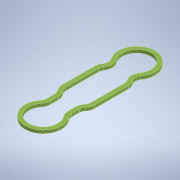
# Autodesk Inventor part: Base Seal
Saved by Autodesk Inventor 2021 (Build 250183000, 183)
## iProperties
Created: 2020-06-02
Part Number: Base Seal
Material: Generic
Document SubType Name: Modeling
Designer: jgray
Density: 1 g/cm^3
Appearance: Default
Author: jgray
Autodesk Inventor part; units mm, degrees
ref_plane "YZ Plane" through (0, 0, 0) normal (1, 0, 0) x (0, 1, 0)
ref_plane "XZ Plane" through (0, 0, 0) normal (0, 1, 0) x (-1, 0, 0)
ref_plane "XY Plane" through (0, 0, 0) normal (0, 0, 1) x (1, 0, 0)
sketch "Sketch1" plane through (0, 0, 0) normal (0, 1, 0) x (-1, 0, 0)
  line L0 (13.9, 33.875) -> (-13.9, 33.875)
  line L1 (-13.9, 33.875) -> (-13.9, -33.875)
  line L2 (-13.9, -33.875) -> (13.9, -33.875)
  line L3 (13.9, -33.875) -> (13.9, 33.875)
  circle A0 centre (9.4, 30.5) radius 1.7
  circle A1 centre (-9.4, 15) radius 1.7
  circle A2 centre (9.4, -15) radius 1.7
  circle A3 centre (-9.4, -15) radius 1.7
  circle A4 centre (-9.4, -30.5) radius 1.7
  circle A5 centre (9.4, -30.5) radius 1.7
  circle A6 centre (9.4, 15) radius 1.7
  circle A7 centre (-9.4, 30.5) radius 1.7
  arc A8 (-3.4662, -17.8593) -> (3.4662, -17.8593) centre (0, -22) ccw
  line L4 (4.7, 5.1) -> (4.7, -10.1)
  arc A9 (2.75, -12.0994) -> (4.7, -10.1) centre (2.7, -10.1) ccw
  arc A10 (-4.7, -10.1) -> (-2.75, -12.0994) centre (-2.7, -10.1) ccw
  line L5 (-4.7, -10.1) -> (-4.7, 5.1)
  line L6 (-2.75, 7.0994) -> (-2.75, 16.3257)
  arc A11 (3.4662, 17.8593) -> (-3.4662, 17.8593) centre (0, 22) ccw
  line L7 (2.75, -12.0994) -> (2.75, -16.3257)
  arc A12 (-5.2039, -18.2745) -> (5.2039, -18.2745) centre (0, -22) ccw
  line L8 (-3.75, 14.4782) -> (-3.75, 11.1034)
  arc A13 (-5.0936, 7.4643) -> (-5.7, 5.8219) centre (-3.1726, 5.8219) ccw
  arc A14 (-5.7, -10.1) -> (-5.1619, -11.8144) centre (-2.7, -10.1) ccw
  arc A15 (5.1619, -11.8144) -> (5.7, -10.1001) centre (2.7, -10.1) ccw
  line L9 (5.7, -10.1001) -> (5.7004, 5.4185)
  arc A16 (5.7004, 5.4185) -> (5.0937, 7.0617) centre (3.1718, 5.4185) ccw
  line L10 (3.75, 10.7009) -> (3.75, 14.4782)
  arc A17 (4.9867, 17.9884) -> (-4.9867, 17.9884) centre (0, 22) ccw
  line L11 (-6.35, 14.4782) -> (-6.35, 11.1034)
  arc A18 (-7.0698, 9.1539) -> (-8.3, 5.8219) centre (-3.1726, 5.8219) ccw
  line L12 (-8.3, 5.8219) -> (-8.3, -10.1)
  arc A19 (-8.3, -10.1) -> (-7.2955, -13.3003) centre (-2.7, -10.1) ccw
  arc A20 (-7.318, -16.761) -> (7.318, -16.761) centre (0, -22) ccw
  arc A21 (7.2955, -13.3003) -> (8.3, -10.1) centre (2.7, -10.1) ccw
  line L13 (8.3, -10.1) -> (8.3, 5.4787)
  arc A22 (8.3, 5.4787) -> (7.0698, 8.7513) centre (3.1718, 5.4185) ccw
  line L14 (6.35, 10.7009) -> (6.35, 14.4782)
  arc A23 (7.0125, 16.3586) -> (-7.0125, 16.3586) centre (0, 22) ccw
  arc A24 (-7.318, -16.761) -> (-7.2955, -13.3003) centre (-9.7573, -15.0147) ccw
  arc A25 (7.2955, -13.3003) -> (7.318, -16.761) centre (9.7573, -15.0147) ccw
  arc A26 (-7.0698, 9.1539) -> (-6.35, 11.1034) centre (-9.35, 11.1034) ccw
  arc A27 (-6.35, 14.4782) -> (-7.0125, 16.3586) centre (-9.35, 14.4782) ccw
  arc A28 (7.0125, 16.3586) -> (6.35, 14.4782) centre (9.35, 14.4782) ccw
  arc A29 (6.35, 10.7009) -> (7.0698, 8.7513) centre (9.35, 10.7009) ccw
  line L15 (-5.7, -10.1) -> (-5.7, 5.8219)
  arc A30 (-5.0936, 7.4643) -> (-5.7, 5.8219) centre (-3.1726, 5.8219) ccw
  arc A31 (-5.0936, 7.4643) -> (-3.75, 11.1034) centre (-9.35, 11.1034) ccw
  line L16 (-3.75, 11.1034) -> (-3.75, 14.4782)
  arc A32 (-3.75, 14.4782) -> (-4.9867, 17.9884) centre (-9.35, 14.4782) ccw
  arc A33 (4.9867, 17.9884) -> (-4.9867, 17.9884) centre (0, 22) ccw
  arc A34 (4.9867, 17.9884) -> (3.75, 14.4782) centre (9.35, 14.4782) ccw
  line L17 (3.75, 14.4782) -> (3.75, 10.7009)
  arc A35 (3.75, 10.7009) -> (5.0937, 7.0617) centre (9.35, 10.7009) ccw
  arc A36 (5.7004, 5.4185) -> (5.0937, 7.0617) centre (3.1718, 5.4185) ccw
  arc A37 (5.1619, -11.8144) -> (5.7, -10.1001) centre (2.7, -10.1) ccw
  arc A38 (5.1619, -11.8144) -> (5.2039, -18.2745) centre (9.7573, -15.0147) ccw
  arc A39 (-5.2039, -18.2745) -> (5.2039, -18.2745) centre (0, -22) ccw
  arc A40 (-5.2039, -18.2745) -> (-5.1619, -11.8144) centre (-9.7573, -15.0147) ccw
  arc A41 (-5.7, -10.1) -> (-5.1619, -11.8144) centre (-2.7, -10.1) ccw
  line L18 (2.75, 16.3257) -> (2.75, 7.0994)
  line L19 (-2.75, -16.3257) -> (-2.75, -12.0994)
  arc A42 (-3.4662, -17.8593) -> (-2.75, -16.3257) centre (-4.75, -16.3257) ccw
  arc A43 (-2.75, 16.3257) -> (-3.4662, 17.8593) centre (-4.75, 16.3257) ccw
  arc A44 (3.4662, 17.8593) -> (2.75, 16.3257) centre (4.75, 16.3257) ccw
  arc A45 (2.75, -16.3257) -> (3.4662, -17.8593) centre (4.75, -16.3257) ccw
  arc A46 (-2.75, 7.0994) -> (-4.7, 5.1) centre (-2.7, 5.1) ccw
  arc A47 (4.7, 5.1) -> (2.75, 7.0994) centre (2.7, 5.1) ccw
  line L20 (0, -33.875) -> (0, 33.875) construction
  arc A48 (-5.95, 14.4782) -> (-6.7008, 16.6094) centre (-9.35, 14.4782) ccw
  line L21 (-5.95, 14.4782) -> (-5.95, 11.1034)
  arc A49 (-6.7658, 8.894) -> (-5.95, 11.1034) centre (-9.35, 11.1034) ccw
  arc A50 (-6.7658, 8.894) -> (-7.9, 5.8219) centre (-3.1726, 5.8219) ccw
  line L22 (-7.9, 5.8219) -> (-7.9, -10.1)
  arc A51 (-7.9, -10.1) -> (-6.9672, -13.0717) centre (-2.7, -10.1) ccw
  arc A52 (-6.9928, -16.9939) -> (-6.9672, -13.0717) centre (-9.7573, -15.0147) ccw
  arc A53 (-6.9928, -16.9939) -> (6.9928, -16.9939) centre (0, -22) ccw
  arc A54 (6.9672, -13.0717) -> (6.9928, -16.9939) centre (9.7573, -15.0147) ccw
  arc A55 (6.9672, -13.0717) -> (7.9, -10.1) centre (2.7, -10.1) ccw
  line L23 (7.9, -10.1) -> (7.9, 5.4763)
  arc A56 (7.9, 5.4763) -> (6.7658, 8.4914) centre (3.1718, 5.4185) ccw
  arc A57 (5.95, 10.7009) -> (6.7658, 8.4914) centre (9.35, 10.7009) ccw
  line L24 (5.95, 10.7009) -> (5.95, 14.4782)
  arc A58 (6.7008, 16.6094) -> (5.95, 14.4782) centre (9.35, 14.4782) ccw
  arc A59 (6.7008, 16.6094) -> (-6.7008, 16.6094) centre (0, 22) ccw
  arc A60 (5.2983, 17.7376) -> (-5.2983, 17.7376) centre (0, 22) ccw
  arc A61 (5.2983, 17.7376) -> (4.15, 14.4782) centre (9.35, 14.4782) ccw
  line L25 (4.15, 10.7009) -> (4.15, 14.4782)
  arc A62 (4.15, 10.7009) -> (5.3977, 7.3216) centre (9.35, 10.7009) ccw
  arc A63 (6.1004, 5.4185) -> (5.3977, 7.3216) centre (3.1718, 5.4185) ccw
  line L26 (6.1004, 5.4185) -> (6.1, -10.1001)
  arc A64 (5.4901, -12.043) -> (6.1, -10.1001) centre (2.7, -10.1) ccw
  arc A65 (5.4901, -12.043) -> (5.5292, -18.0417) centre (9.7573, -15.0147) ccw
  arc A66 (-5.5292, -18.0417) -> (5.5292, -18.0417) centre (0, -22) ccw
  arc A67 (-5.5292, -18.0417) -> (-5.4901, -12.043) centre (-9.7573, -15.0147) ccw
  arc A68 (-6.1, -10.1) -> (-5.4901, -12.043) centre (-2.7, -10.1) ccw
  line L27 (-6.1, -10.1) -> (-6.1, 5.8219)
  arc A69 (-5.3976, 7.7242) -> (-6.1, 5.8219) centre (-3.1726, 5.8219) ccw
  arc A70 (-5.3976, 7.7242) -> (-4.15, 11.1034) centre (-9.35, 11.1034) ccw
  line L28 (-4.15, 14.4782) -> (-4.15, 11.1034)
  arc A71 (-4.15, 14.4782) -> (-5.2983, 17.7376) centre (-9.35, 14.4782) ccw
  point P0 (0, 0)
  point P1 (0, 0)
  point P2 (-6.35, 15.6221)
  point P3 (-6.35, 9.8461)
  point P4 (6.35, 9.4436)
  point P5 (6.35, 15.6221)
  point P6 (-7.3624, -13.3004)
  point P7 (-5.7039, -14.8852)
  point P8 (-5.7004, -15.0354)
  point P9 (-7.2703, -16.695)
  point P10 (7.2703, -16.695)
  point P11 (5.7004, -15.0354)
  point P12 (5.7039, -14.8852)
  point P13 (7.3624, -13.3004)
  point P14 (6.35, 13.663)
  point P15 (7.2703, 16.695)
  point P16 (-7.2703, 16.695)
  point P17 (-6.35, 13.663)
  point P18 (-5.7, 5.8219)
  point P19 (5.3977, 7.3216)
  point P20 (5.5292, -18.0417)
  point P21 (-5.4901, -12.043)
  point P22 (-5.2983, 17.7376)
  point P23 (4.15, 14.4782)
  dimension "d0" = 1
  dimension "d1" = 1
  dimension "d2" = 3
  dimension "d3" = 2.6
  dimension "d4" = 8.3
  dimension "d5" = 1
  dimension "d6" = 0.4
  dimension "d7" = 0.4
  dimension "d8" = 0.4
  dimension "d9" = 0.4
  dimension "d10" = 0.4
  dimension "d11" = 0.4
  dimension "d12" = 0.4
  dimension "d13" = 0.4
  dimension "d14" = 0.4
  dimension "d15" = 0.4
  dimension "d16" = 0.4
  dimension "d17" = 0.4
  dimension "d18" = 0.4
  dimension "d19" = 0.4
  dimension "d20" = 0.4
  constraints: 132 point on circle, 72 centre point, 58 end point, 18 tangent, 6 parallel, 5 equal radius, 4 point on line, 2 midpoint, 1 coincident, 32 other
  measures "d0" radial gap between concentric circles of A12 A8
  measures "d1" radial gap between concentric circles of A11 A17
  measures "d2" radius of A24
  measures "d3" distance between parallel lines of L12 L15
  measures "d4" distance from line of L13 point (0, 0)
  measures "d5" distance between parallel lines of L8 L6
  measures "d6" radial gap between concentric circles of A23 A59
  measures "d7" radial gap between concentric circles of A17 A60
  measures "d8" radial gap between concentric circles of A34 A61
  measures "d9" distance between parallel lines of L10 L25
  measures "d10" radial gap between concentric circles of A35 A62
  measures "d11" radial gap between concentric circles of A16 A63
  measures "d12" radial gap between concentric circles of A15 A64
  measures "d13" radial gap between concentric circles of A38 A65
  measures "d14" radial gap between concentric circles of A39 A66
  measures "d15" radial gap between concentric circles of A40 A67
  measures "d16" radial gap between concentric circles of A14 A68
  measures "d17" distance between parallel lines of L15 L27
  measures "d18" radial gap between concentric circles of A31 A70
  measures "d19" distance between parallel lines of L8 L28
  measures "d20" radial gap between concentric circles of A32 A71
extrude "Extrusion1" add sketch "Sketch1" along normal blind 1.5 contours A48 A59 A58 L24 A57 A56 L23 A55 A54 A53 A52 A51 L22 A50 A49 L21
body "Solid1"
